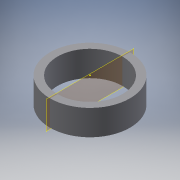
# Autodesk Inventor part: Bearing 608 Outer Race
Saved by Autodesk Inventor 2018 (Build 220112000, 112)
## iProperties
Created: 2017-09-15
Part Number: Bearing 608 Outer Race
Material: Generic
Document SubType Name: Modeling
Designer: Rus
Density: 1 g/cm^3
Appearance: Default
Author: Rus
Autodesk Inventor part; units mm, degrees
ref_plane "YZ Plane" through (0, 0, 0) normal (1, 0, 0) x (0, 1, 0)
ref_plane "XZ Plane" through (0, 0, 0) normal (0, 1, 0) x (-1, 0, 0)
ref_plane "XY Plane" through (0, 0, 0) normal (0, 0, 1) x (1, 0, 0)
sketch "Sketch1" plane through (0, 0, 0) normal (0, 0, 1) x (1, 0, 0)
  circle A0 centre (2.8404, 0) radius 8.95
  circle A1 centre (2.8404, 0) radius 11
  point P0 (0, 0)
  dimension "d0" = 17.9
  dimension "d1" = 22
  constraints: 2 centre point, 2 coincident
  measures "d0" diameter of A0
  measures "d1" diameter of A1
extrude "Extrusion1" add sketch "Sketch1" against normal blind 7
ref_plane "Work Plane1" through (2.8404, 6.05, 0) normal (1, 0, 0) x (0, 0, -1)
sketch "Sketch2" plane through (2.8404, 6.05, 0) normal (1, 0, 0) x (0, 0, -1)
  point P0 (0, -6.05)
body "Solid1"
